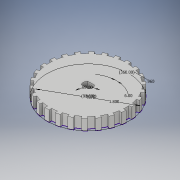
# Autodesk Inventor part: Wheel
Saved by Autodesk Inventor 2019 (Build 230136000, 136)
## iProperties
Created: 2019-10-19
Part Number: Wheel
Material: Generic
Document SubType Name: Modeling
Designer: Bryce V
Density: 1 g/cm^3
Appearance: Default
Author: Bryce V
## iProperties of the stored document Wheel_3DPrint.ipt
Created: 2019-10-19
Part Number: Wheel_3DPrint
Material: Generic
Document SubType Name: Modeling
Designer: Bryce V
Density: 1 g/cm^3
Appearance: Default
Author: Bryce V
Autodesk Inventor part; units mm, degrees
ref_plane "YZ Plane" through (0, 0, 0) normal (1, 0, 0) x (0, 1, 0)
ref_plane "XZ Plane" through (0, 0, 0) normal (0, 1, 0) x (-1, 0, 0)
ref_plane "XY Plane" through (0, 0, 0) normal (0, 0, 1) x (1, 0, 0)
sketch "Sketch1" plane through (0, 0, 0) normal (0, 1, 0) x (-1, 0, 0)
  circle A0 centre (0, 0) radius 22.86
  arc A1 (-1.2762, -24.3506) -> (1.2762, -24.3506) centre (0, 0) ccw
  line L0 (0, 0) -> (1.2762, -24.3506) construction
  line L1 (0, 0) -> (24.384, 0) construction
  line L2 (0, 0) -> (-1.2762, -24.3506) construction
  line L3 (1.2762, -24.3506) -> (1.1964, -22.8287)
  line L4 (-1.2762, -24.3506) -> (-1.1964, -22.8287)
  line L5 (0, 0) -> (7.0666, -23.3376) construction
  line L6 (7.0666, -23.3376) -> (6.6249, -21.879)
  arc A2 (4.5884, -23.9484) -> (7.0666, -23.3376) centre (0, 0) ccw
  line L7 (0, 0) -> (4.5884, -23.9484) construction
  line L8 (4.5884, -23.9484) -> (4.3016, -22.4516)
  circle A3 centre (0, 0) radius 22.86
  line L9 (0, 0) -> (12.4463, -20.9683) construction
  line L10 (12.4463, -20.9683) -> (11.6684, -19.6578)
  arc A4 (10.1863, -22.1544) -> (12.4463, -20.9683) centre (0, 0) ccw
  line L11 (0, 0) -> (10.1863, -22.1544) construction
  line L12 (10.1863, -22.1544) -> (9.5497, -20.7698)
  circle A5 centre (0, 0) radius 22.86
  line L13 (0, 0) -> (17.1026, -17.3804) construction
  line L14 (17.1026, -17.3804) -> (16.0337, -16.2941)
  arc A6 (15.1922, -19.0729) -> (17.1026, -17.3804) centre (0, 0) ccw
  line L15 (0, 0) -> (15.1922, -19.0729) construction
  line L16 (15.1922, -19.0729) -> (14.2427, -17.8809)
  circle A7 centre (0, 0) radius 22.86
  line L17 (0, 0) -> (20.7651, -12.7824) construction
  line L18 (20.7651, -12.7824) -> (19.4673, -11.9835)
  arc A8 (19.3152, -14.883) -> (20.7651, -12.7824) centre (0, 0) ccw
  line L19 (0, 0) -> (19.3152, -14.883) construction
  line L20 (19.3152, -14.883) -> (18.108, -13.9528)
  circle A9 centre (0, 0) radius 22.86
  line L21 (0, 0) -> (23.2207, -7.4416) construction
  line L22 (23.2207, -7.4416) -> (21.7694, -6.9765)
  arc A10 (22.3157, -9.8281) -> (23.2207, -7.4416) centre (0, 0) ccw
  line L23 (0, 0) -> (22.3157, -9.8281) construction
  line L24 (22.3157, -9.8281) -> (20.9209, -9.2138)
  circle A11 centre (0, 0) radius 22.86
  line L25 (0, 0) -> (24.3269, -1.6683) construction
  line L26 (24.3269, -1.6683) -> (22.8064, -1.564)
  arc A12 (24.0192, -4.202) -> (24.3269, -1.6683) centre (0, 0) ccw
  line L27 (0, 0) -> (24.0192, -4.202) construction
  line L28 (24.0192, -4.202) -> (22.518, -3.9394)
  circle A13 centre (0, 0) radius 22.86
  line L29 (0, 0) -> (24.0192, 4.202) construction
  line L30 (24.0192, 4.202) -> (22.518, 3.9394)
  arc A14 (24.3269, 1.6683) -> (24.0192, 4.202) centre (0, 0) ccw
  line L31 (0, 0) -> (24.3269, 1.6683) construction
  line L32 (24.3269, 1.6683) -> (22.8064, 1.564)
  circle A15 centre (0, 0) radius 22.86
  line L33 (0, 0) -> (22.3157, 9.8281) construction
  line L34 (22.3157, 9.8281) -> (20.9209, 9.2138)
  arc A16 (23.2207, 7.4416) -> (22.3157, 9.8281) centre (0, 0) ccw
  line L35 (0, 0) -> (23.2207, 7.4416) construction
  line L36 (23.2207, 7.4416) -> (21.7694, 6.9765)
  circle A17 centre (0, 0) radius 22.86
  line L37 (0, 0) -> (19.3152, 14.883) construction
  line L38 (19.3152, 14.883) -> (18.108, 13.9528)
  arc A18 (20.7651, 12.7824) -> (19.3152, 14.883) centre (0, 0) ccw
  line L39 (0, 0) -> (20.7651, 12.7824) construction
  line L40 (20.7651, 12.7824) -> (19.4673, 11.9835)
  circle A19 centre (0, 0) radius 22.86
  line L41 (0, 0) -> (15.1922, 19.0729) construction
  line L42 (15.1922, 19.0729) -> (14.2427, 17.8809)
  arc A20 (17.1026, 17.3804) -> (15.1922, 19.0729) centre (0, 0) ccw
  line L43 (0, 0) -> (17.1026, 17.3804) construction
  line L44 (17.1026, 17.3804) -> (16.0337, 16.2941)
  circle A21 centre (0, 0) radius 22.86
  line L45 (0, 0) -> (10.1863, 22.1544) construction
  line L46 (10.1863, 22.1544) -> (9.5497, 20.7698)
  arc A22 (12.4463, 20.9683) -> (10.1863, 22.1544) centre (0, 0) ccw
  line L47 (0, 0) -> (12.4463, 20.9683) construction
  line L48 (12.4463, 20.9683) -> (11.6684, 19.6578)
  circle A23 centre (0, 0) radius 22.86
  line L49 (0, 0) -> (4.5884, 23.9484) construction
  line L50 (4.5884, 23.9484) -> (4.3016, 22.4516)
  arc A24 (7.0666, 23.3376) -> (4.5884, 23.9484) centre (0, 0) ccw
  line L51 (0, 0) -> (7.0666, 23.3376) construction
  line L52 (7.0666, 23.3376) -> (6.6249, 21.879)
  circle A25 centre (0, 0) radius 22.86
  line L53 (0, 0) -> (-1.2762, 24.3506) construction
  line L54 (-1.2762, 24.3506) -> (-1.1964, 22.8287)
  arc A26 (1.2762, 24.3506) -> (-1.2762, 24.3506) centre (0, 0) ccw
  line L55 (0, 0) -> (1.2762, 24.3506) construction
  line L56 (1.2762, 24.3506) -> (1.1964, 22.8287)
  circle A27 centre (0, 0) radius 22.86
  line L57 (0, 0) -> (-7.0666, 23.3376) construction
  line L58 (-7.0666, 23.3376) -> (-6.6249, 21.879)
  arc A28 (-4.5884, 23.9484) -> (-7.0666, 23.3376) centre (0, 0) ccw
  line L59 (0, 0) -> (-4.5884, 23.9484) construction
  line L60 (-4.5884, 23.9484) -> (-4.3016, 22.4516)
  circle A29 centre (0, 0) radius 22.86
  line L61 (0, 0) -> (-12.4463, 20.9683) construction
  line L62 (-12.4463, 20.9683) -> (-11.6684, 19.6578)
  arc A30 (-10.1863, 22.1544) -> (-12.4463, 20.9683) centre (0, 0) ccw
  line L63 (0, 0) -> (-10.1863, 22.1544) construction
  line L64 (-10.1863, 22.1544) -> (-9.5497, 20.7698)
  circle A31 centre (0, 0) radius 22.86
  line L65 (0, 0) -> (-17.1026, 17.3804) construction
  line L66 (-17.1026, 17.3804) -> (-16.0337, 16.2941)
  arc A32 (-15.1922, 19.0729) -> (-17.1026, 17.3804) centre (0, 0) ccw
  line L67 (0, 0) -> (-15.1922, 19.0729) construction
  line L68 (-15.1922, 19.0729) -> (-14.2427, 17.8809)
  circle A33 centre (0, 0) radius 22.86
  line L69 (0, 0) -> (-20.7651, 12.7824) construction
  line L70 (-20.7651, 12.7824) -> (-19.4673, 11.9835)
  arc A34 (-19.3152, 14.883) -> (-20.7651, 12.7824) centre (0, 0) ccw
  line L71 (0, 0) -> (-19.3152, 14.883) construction
  line L72 (-19.3152, 14.883) -> (-18.108, 13.9528)
  circle A35 centre (0, 0) radius 22.86
  line L73 (0, 0) -> (-23.2207, 7.4416) construction
  line L74 (-23.2207, 7.4416) -> (-21.7694, 6.9765)
  arc A36 (-22.3157, 9.8281) -> (-23.2207, 7.4416) centre (0, 0) ccw
  line L75 (0, 0) -> (-22.3157, 9.8281) construction
  line L76 (-22.3157, 9.8281) -> (-20.9209, 9.2138)
  circle A37 centre (0, 0) radius 22.86
  line L77 (0, 0) -> (-24.3269, 1.6683) construction
  line L78 (-24.3269, 1.6683) -> (-22.8064, 1.564)
  arc A38 (-24.0192, 4.202) -> (-24.3269, 1.6683) centre (0, 0) ccw
  line L79 (0, 0) -> (-24.0192, 4.202) construction
  line L80 (-24.0192, 4.202) -> (-22.518, 3.9394)
  circle A39 centre (0, 0) radius 22.86
  line L81 (0, 0) -> (-24.0192, -4.202) construction
  line L82 (-24.0192, -4.202) -> (-22.518, -3.9394)
  arc A40 (-24.3269, -1.6683) -> (-24.0192, -4.202) centre (0, 0) ccw
  line L83 (0, 0) -> (-24.3269, -1.6683) construction
  line L84 (-24.3269, -1.6683) -> (-22.8064, -1.564)
  circle A41 centre (0, 0) radius 22.86
  line L85 (0, 0) -> (-22.3157, -9.8281) construction
  line L86 (-22.3157, -9.8281) -> (-20.9209, -9.2138)
  arc A42 (-23.2207, -7.4416) -> (-22.3157, -9.8281) centre (0, 0) ccw
  line L87 (0, 0) -> (-23.2207, -7.4416) construction
  line L88 (-23.2207, -7.4416) -> (-21.7694, -6.9765)
  circle A43 centre (0, 0) radius 22.86
  line L89 (0, 0) -> (-19.3152, -14.883) construction
  line L90 (-19.3152, -14.883) -> (-18.108, -13.9528)
  arc A44 (-20.7651, -12.7824) -> (-19.3152, -14.883) centre (0, 0) ccw
  line L91 (0, 0) -> (-20.7651, -12.7824) construction
  line L92 (-20.7651, -12.7824) -> (-19.4673, -11.9835)
  circle A45 centre (0, 0) radius 22.86
  line L93 (0, 0) -> (-15.1922, -19.0729) construction
  line L94 (-15.1922, -19.0729) -> (-14.2427, -17.8809)
  arc A46 (-17.1026, -17.3804) -> (-15.1922, -19.0729) centre (0, 0) ccw
  line L95 (0, 0) -> (-17.1026, -17.3804) construction
  line L96 (-17.1026, -17.3804) -> (-16.0337, -16.2941)
  circle A47 centre (0, 0) radius 22.86
  line L97 (0, 0) -> (-10.1863, -22.1544) construction
  line L98 (-10.1863, -22.1544) -> (-9.5497, -20.7698)
  arc A48 (-12.4463, -20.9683) -> (-10.1863, -22.1544) centre (0, 0) ccw
  line L99 (0, 0) -> (-12.4463, -20.9683) construction
  line L100 (-12.4463, -20.9683) -> (-11.6684, -19.6578)
  circle A49 centre (0, 0) radius 22.86
  line L101 (0, 0) -> (-4.5884, -23.9484) construction
  line L102 (-4.5884, -23.9484) -> (-4.3016, -22.4516)
  arc A50 (-7.0666, -23.3376) -> (-4.5884, -23.9484) centre (0, 0) ccw
  line L103 (0, 0) -> (-7.0666, -23.3376) construction
  line L104 (-7.0666, -23.3376) -> (-6.6249, -21.879)
  circle A51 centre (0, 0) radius 22.86
  line L105 (0, 0) -> (0, -1.905)
  line L106 (0, 0) -> (1.905, 0) construction
  line L107 (0, -1.905) -> (-2.0439, -1.905)
  line L108 (2.0439, 1.905) -> (-2.0439, 1.905)
  line L109 (-2.0439, -1.905) -> (2.0439, -1.905)
  line L110 (2.0439, 1.905) -> (-2.0439, -1.905) construction
  line L111 (-2.0439, 1.905) -> (2.0439, -1.905) construction
  arc A52 (2.0439, -1.905) -> (2.0439, 1.905) centre (0, 0) ccw
  arc A53 (-2.0439, 1.905) -> (-2.0439, -1.905) centre (0, 0) ccw
  dimension "d0" = 45.72
  dimension "d1" = 24.384
  dimension "d2" = 87
  dimension "d3" = 6
  dimension "d6" = 360
  dimension "d11" = 1.905
  dimension "d12" = 90
  dimension "d13" = 90
  constraints: 224 end point, 108 point on circle, 54 centre point, 52 point on line, 28 coincident, 3 horizontal, 2 equal length, 2 midpoint, 1 parallel, 1 vertical, 313 other
  measures "d0" diameter of A0
  measures "d1" radius of A1
  measures "d2" angle of L0 L1
  measures "d3" angle of L2 L0
  measures "d11" distance of L105.start L105.end
  measures "d12" angle of L105 L106
  measures "d13" angle of L105 L107
extrude "Extrusion1" add sketch "Sketch1" along normal blind 6.35 contours A0 | A0 L30 A14 L32 | L26 A12 L28 A0 | A0 L34 A16 L36 | L22 A10 L24 A0 | A0 L38 A18 L40 | L18 A8 L20 A0 | A0 L42 A20 L44 | L14 A6 L16 A0 | A0 L46 A22 L48 | L10 A4 L12 A0 | A0 L50 A24 L52 | L6 A2 L8 A0 | A0 L54 A26 L56 | L3 A1 L4 A0 | A0 L58 A28 L60 | L102 A50 L104 A0 | A0 L62 A30 L64 | L98 A48 L100 A0 | A0 L66 A32 L68 | L94 A46 L96 A0 | A0 L70 A34 L72 | L90 A44 L92 A0 | A0 L74 A36 L76 | L86 A42 L88 A0 | A0 L78 A38 L80 | L82 A40 L84 A0 | L107 A53 L108 A52 L109
extrude "Extrusion2" cut sketch "Sketch1" along normal blind 9.525 contours L107 A53 L108 A52 L109
body "Solid1"
